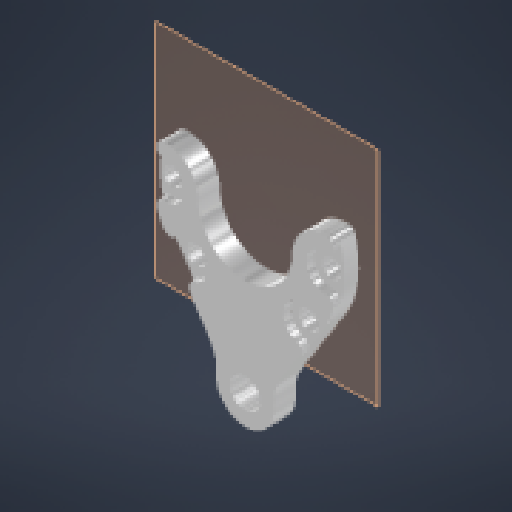
# Autodesk Inventor part: Slider_crank_horn_v2_2025
Saved by Autodesk Inventor 2024.3 (Build 283343000, 343)
## iProperties
Created: 2024-01-23
Part Number: Slider_crank_horn_v2_2025
Material: 알루미늄 6061
Document SubType Name: Modeling
Designer: ASUS
Density: 2.7 g/cm^3
Appearance: 알루미늄 - 평지
Author: ASUS
Autodesk Inventor part; units mm, degrees
(part 1 of 2)
ref_plane "YZ Plane" through (0, 0, 0) normal (1, 0, 0) x (0, 1, 0)
ref_plane "XZ Plane" through (0, 0, 0) normal (0, 1, 0) x (-1, 0, 0)
ref_plane "XY Plane" through (0, 0, 0) normal (0, 0, 1) x (1, 0, 0)
ref_plane "작업 평면1" through (0, 0, 0) normal (0, 0, 1) x (1, 0, 0)
sketch "스케치1" plane through (0, 0, 0) normal (0, 0, 1) x (1, 0, 0)
  circle A0 centre (-11, 0) radius 1.25 projected
  circle A1 centre (11, 0) radius 1.25 projected
  circle A2 centre (7.7782, -7.7782) radius 1.25 projected
  circle A3 centre (-7.7782, 7.7782) radius 1.25 projected
  circle A4 centre (-7.7782, -7.7782) radius 1.25 projected
  circle A5 centre (7.7782, 7.7782) radius 1.25 projected
  circle A6 centre (0, -11) radius 1.25 projected
  circle A7 centre (0, 11) radius 1.25 projected
  circle A8 centre (0, 0) radius 14 projected
  circle A9 centre (0, 0) radius 5 projected
  line L0 (-17, -38.65) -> (-17, -41.35) projected
  line L1 (17, -38.65) -> (17, -41.35) projected
  line L2 (-17, -40) -> (17, -40)
  line L3 (0, -40) -> (0, 0)
  circle A10 centre (0, -20) radius 2.75
  line L4 (-7.7782, -7.7782) -> (0, -20) construction
  line L5 (-11.1527, -9.9258) -> (-3.3746, -22.1476)
  line L6 (3.3746, -17.8524) -> (-4.4036, -5.6305)
  arc A11 (-4.4036, -5.6305) -> (-11.1527, -9.9258) centre (-7.7782, -7.7782) ccw
  arc A12 (-3.3746, -22.1476) -> (3.3746, -17.8524) centre (0, -20) ccw
  line L7 (0, -20) -> (7.7782, -7.7782) construction
  line L8 (-3.3746, -17.8524) -> (4.4036, -5.6305)
  line L9 (11.1527, -9.9258) -> (3.3746, -22.1476)
  arc A13 (-3.3746, -17.8524) -> (3.3746, -22.1476) centre (0, -20) ccw
  arc A14 (11.1527, -9.9258) -> (4.4036, -5.6305) centre (7.7782, -7.7782) ccw
  circle A15 centre (0, 0) radius 7
  circle A16 centre (-7.7782, -7.7782) radius 1.35
  circle A17 centre (0, -11) radius 1.85
  circle A18 centre (7.7782, -7.7782) radius 1.35
  circle A19 centre (0, 0) radius 11
  circle A20 centre (0, 0) radius 9
  circle A21 centre (0, 0) radius 11
  circle A22 centre (0, 0) radius 13
  line L10 (7.7782, -7.7782) -> (0, -20) construction
  line L11 (6.0909, -6.7044) -> (-1.6873, -18.9262)
  line L12 (1.6873, -21.0738) -> (12.1403, -4.6491)
  arc A23 (9.4655, -8.852) -> (6.0909, -6.7044) centre (7.7782, -7.7782) ccw
  arc A24 (-1.6873, -18.9262) -> (1.6873, -21.0738) centre (0, -20) ccw
  line L13 (0, -20) -> (-7.7782, -7.7782) construction
  line L14 (1.6873, -18.9262) -> (-6.0909, -6.7044)
  line L15 (-12.1403, -4.6491) -> (-1.6873, -21.0738)
  arc A25 (-1.6873, -21.0738) -> (1.6873, -18.9262) centre (0, -20) ccw
  arc A26 (-6.0909, -6.7044) -> (-9.4655, -8.852) centre (-7.7782, -7.7782) ccw
  point P0 (-3.8891, -13.8891)
  point P1 (3.8891, -13.8891)
  point P2 (4.9497, -4.9497)
  point P3 (-4.9497, -4.9497)
  point P4 (0.2013, -12.2337)
  point P5 (0, -12.5499)
  point P6 (-0.2013, -12.2337)
  point P7 (3.8891, -13.8891)
  point P8 (-3.8891, -13.8891)
  point P9 (-3.5472, -18.1514)
  point P10 (-3.3746, -22.1476)
  point P11 (3.5472, -18.1514)
  dimension "d0" = 5.5
  dimension "d1" = 8
  dimension "d2" = 2.7
  dimension "d3" = 3.7
  dimension "d4" = 2.7
  dimension "d7" = 2
  dimension "d8" = 2
  dimension "d9" = 2
  dimension "d10" = 4
  dimension "d11" = 4
  constraints: 36 end point, 18 point on circle, 17 tangent, 16 centre point, 8 midpoint, 5 coincident, 4 parallel, 2 collinear, 2 point on line, 1 concentric, 1 vertical, 3 other
  measures "d0" diameter of A10
  measures "d1" diameter of A12
  measures "d2" diameter of A16
  measures "d3" diameter of A17
  measures "d4" diameter of A18
  measures "d8" radial gap between concentric circles of A20 A21
  measures "d9" radial gap between concentric circles of A21 A22
  measures "d10" diameter of A24
  measures "d11" diameter of A26
extrude "돌출1" add sketch "스케치1" along normal blind 5 contours A0 A19 A3 A7 A5 A1 A14 A20 A11 | A0 A19 A11 L15 A22 L12 A14 A1 A5 A7 A3 | A19 A26 L15 A11 | A11 A20 A26 A19 | A26 L14 A19 A16 | A19 A16 L14 A22 L15 A26 | A20 L6 A17 A19 L14 A26 | A14 A19 A23 A20 | A20 L3 A17 L6 | A22 L14 A8 L15 | A20 L8 A17 L3 | A14 L12 A23 A19 | A23 L11 A19 A17 L8 A20 | A23 A19 A18 L11 | A17 L3 A6 L6 | L6 A6 A19 A17 | A19 A17 L8 A22 L14 | A8 L14 L8 A13 L15 | A22 L8 A8 L14 | A17 L8 A6 L3 | A23 L12 A22 L11 A19 A18 | A19 A6 L6 L8 A17 | A8 L8 L14 | L15 A10 L3 A12 A13 | A13 L8 L14 L11 A10 L15 | A22 L3 A8 L8 | L8 A17 L3 A22 | A17 A19 A6 L8 | L11 A22 L6 A17 A19 | L8 L3 A17 | L12 A12 L6 L11 A8 | A8 L11 A22 L12 | A8 L3 L14 L8 | L3 A10 L12 A12 | A22 L6 A8 L3 | L3 A17 L6 A22 | A17 L6 L8 A6 A19 | L11 A8 L6 A22 | A6 L3 L6 | L6 A17 L3 | L3 A6 L8 | L11 L6 A8 | L12 A10 L14 L11 L6 A12 | A8 L6 L11 L3 | L14 A10 L3 | L3 A10 L11
sketch "스케치2" plane through (0, 0, 5) normal (0, 0, 1) x (1, 0, 0)
  circle A0 centre (0, -11) radius 1.25 projected
  circle A1 centre (7.7782, -7.7782) radius 1.35 projected
  circle A2 centre (-11, 0) radius 1.25 projected
  circle A3 centre (-7.7782, -7.7782) radius 1.35 projected
  circle A4 centre (0, -20) radius 2.75 projected
  circle A5 centre (0, 0) radius 9 projected
  circle A6 centre (-7.7782, 7.7782) radius 1.25 projected
  circle A7 centre (0, 11) radius 1.25 projected
  circle A8 centre (7.7782, 7.7782) radius 1.25 projected
  circle A9 centre (11, 0) radius 1.25 projected
  arc A10 (12.1403, -4.6491) -> (-12.1403, -4.6491) centre (0, 0) ccw projected
  line L0 (-12.1403, -4.6491) -> (-3.5472, -18.1514) projected
  arc A11 (-3.5472, -18.1514) -> (3.5472, -18.1514) centre (0, -20) ccw projected
  line L1 (3.5472, -18.1514) -> (12.1403, -4.6491) projected
  circle A12 centre (0, 0) radius 12.7381
  line L2 (3.5472, -18.1514) -> (12.1403, -4.6491) projected
  point P0 (-10.7464, -6.8392)
  point P1 (10.7464, -6.8392)
  constraints: 1 centre point, 1 coincident, 1 tangent
extrude "돌출2" cut sketch "스케치2" against normal through all contours L1 A12 L0 A10
sketch "스케치3" plane through (0, 0, 5) normal (0, 0, 1) x (1, 0, 0)
  circle A0 centre (7.7782, -7.7782) radius 1.35 projected
  circle A1 centre (7.7782, -7.7782) radius 2.5
  circle A2 centre (11, 0) radius 2.5
  circle A3 centre (7.7782, 7.7782) radius 2.5
  circle A4 centre (0, 11) radius 2.5
  circle A5 centre (-7.7782, 7.7782) radius 2.5
  circle A6 centre (-11, 0) radius 2.5
  circle A7 centre (-7.7782, -7.7782) radius 2.5
  circle A8 centre (0, -11) radius 2.5
  point P0 (0, 0)
  dimension "d14" = 5
  dimension "d17" = 360
  constraints: 8 centre point, 1 coincident, 17 other
  measures "d14" diameter of A1
extrude "돌출3" cut sketch "스케치3" against normal blind 2 contours A0 | A1 | A2 | A3 | A4 | A5 | A6 | A7 | A8
fillet "모깎기1" radius 1 30 edges at (5.335, -7.2483, 4) (8.6601, -10.1175, 4) (7.2483, -5.335, 4) (10.2708, -7.5865, 4) (12.5914, -1.9281, 4) (12.5914, 1.9281, 4) (8.8977, 1.3529, 4) (8.8977, -1.3529, 4) (1.3529, -8.8977, 4) (-1.3529, -8.8977, 4) (-5.335, -7.2483, 4) (-7.2483, -5.335, 4) (-8.8977, -1.3529, 4) (-8.6601, -10.1175, 4) (-10.2708, -7.5865, 4) (10.2668, 7.5401, 4) (7.2483, 5.335, 4) (5.335, 7.2483, 4) (7.5401, 10.2668, 4) (1.9281, 12.5914, 4) (-1.3529, 8.8977, 4) (-1.9281, 12.5914, 4) (1.3529, 8.8977, 4) (-5.335, 7.2483, 4) (-7.2483, 5.335, 4) (-7.5401, 10.2668, 4) (-10.2668, 7.5401, 4) (-12.5914, 1.9281, 4) (-8.8977, 1.3529, 4) (-12.5914, -1.9281, 4)
fillet "모깎기2" radius 5 2 edges at (-3.5472, -18.1514, 2.5) (3.5472, -18.1514, 2.5)
sketch "스케치4" plane through (0, 0, 0) normal (0, 0, -1) x (-1, 0, 0)
  arc A0 (10.7464, -6.8392) -> (-10.7464, -6.8392) centre (0, 0) ccw projected
  line L0 (-4.7245, -16.3015) -> (-10.7464, -6.8392) projected
  arc A1 (-3.9745, -19.5493) -> (-4.7245, -16.3015) centre (-8.9427, -18.986) ccw projected
  arc A2 (-3.9745, -19.5493) -> (3.9745, -19.5493) centre (0, -20) ccw projected
  arc A3 (4.7245, -16.3015) -> (3.9745, -19.5493) centre (8.9427, -18.986) ccw projected
  line L1 (10.7464, -6.8392) -> (4.7245, -16.3015) projected
  circle A4 centre (0, -11) radius 1.25 projected
  circle A5 centre (-7.7782, -7.7782) radius 1.35 projected
  circle A6 centre (11, 0) radius 1.25 projected
  circle A7 centre (7.7782, -7.7782) radius 1.35 projected
  circle A8 centre (0, -20) radius 2.75 projected
  circle A9 centre (0, 0) radius 9 projected
  circle A10 centre (7.7782, 7.7782) radius 1.25 projected
  circle A11 centre (0, 11) radius 1.25 projected
  circle A12 centre (-7.7782, 7.7782) radius 1.25 projected
  circle A13 centre (-11, 0) radius 1.25 projected
  circle A14 centre (0, -20) radius 2 projected
  circle A15 centre (0, -20) radius 3 projected
ref_plane "작업 평면2" through (-3.18, -23.18, 4) normal (0, 0, -1) x (-0.0608395, 0.9981476, 0)
extrude "돌출4" add sketch "스케치4" against normal up to surface (4 mm away) contours A8
sketch "스케치5" plane through (0, 0, 0) normal (0, 0, -1) x (-1, 0, 0)
  circle A0 centre (0, -20) radius 2 projected
  arc A1 (10.7464, -6.8392) -> (-10.7464, -6.8392) centre (0, 0) ccw projected
  line L0 (-4.7245, -16.3015) -> (-10.7464, -6.8392) projected
  arc A2 (-3.9745, -19.5493) -> (-4.7245, -16.3015) centre (-8.9427, -18.986) ccw projected
  arc A3 (-3.9745, -19.5493) -> (3.9745, -19.5493) centre (0, -20) ccw projected
  arc A4 (4.7245, -16.3015) -> (3.9745, -19.5493) centre (8.9427, -18.986) ccw projected
  line L1 (10.7464, -6.8392) -> (4.7245, -16.3015) projected
  circle A5 centre (0, -11) radius 1.25 projected
  circle A6 centre (-7.7782, -7.7782) radius 1.35 projected
  circle A7 centre (11, 0) radius 1.25 projected
  circle A8 centre (7.7782, -7.7782) radius 1.35 projected
  circle A9 centre (0, 0) radius 9 projected
  circle A10 centre (7.7782, 7.7782) radius 1.25 projected
  circle A11 centre (0, 11) radius 1.25 projected
  circle A12 centre (-7.7782, 7.7782) radius 1.25 projected
  circle A13 centre (-11, 0) radius 1.25 projected
  circle A14 centre (0, -20) radius 1.75
  dimension "d25" = 3.5
  constraints: 1 centre point, 1 coincident
  measures "d25" diameter of A14
extrude "돌출5" add sketch "스케치5" against normal up to surface (4 mm away) contours A0
sketch "스케치6" plane through (0, 0, 3) normal (0, 0, 1) x (1, 0, 0)
  arc A0 (-4.0295, 8.0475) -> (-8.0475, 4.0295) centre (0, 0) ccw projected
  arc A1 (-5.4204, 8.6093) -> (-4.0295, 8.0475) centre (-4.4772, 8.9417) ccw projected
  arc A2 (-5.4204, 8.6093) -> (-6.1176, 9.647) centre (-7.7782, 7.7782) ccw projected
  arc A3 (-5.9179, 11.28) -> (-6.1176, 9.647) centre (-5.4533, 10.3945) ccw projected
  arc A4 (-5.9179, 11.28) -> (-11.28, 5.9179) centre (0, 0) ccw projected
  arc A5 (-9.647, 6.1176) -> (-11.28, 5.9179) centre (-10.3945, 5.4533) ccw projected
  arc A6 (-9.647, 6.1176) -> (-8.6093, 5.4204) centre (-7.7782, 7.7782) ccw projected
  arc A7 (-8.0475, 4.0295) -> (-8.6093, 5.4204) centre (-8.9417, 4.4772) ccw projected
  circle A8 centre (-7.7782, 7.7782) radius 1.25 projected
  circle A9 centre (0, 11) radius 1.25 projected
  arc A10 (2.8412, 8.5398) -> (-2.8412, 8.5398) centre (0, 0) ccw projected
  arc A11 (2.2549, 9.9205) -> (2.8412, 8.5398) centre (3.1569, 9.4886) ccw projected
  arc A12 (2.2549, 9.9205) -> (2.4957, 11.1472) centre (0, 11) ccw projected
  arc A13 (3.7916, 12.1608) -> (2.4957, 11.1472) centre (3.4939, 11.2061) ccw projected
  arc A14 (3.7916, 12.1608) -> (-3.7916, 12.1608) centre (0, 0) ccw projected
  arc A15 (-2.4957, 11.1472) -> (-3.7916, 12.1608) centre (-3.4939, 11.2061) ccw projected
  arc A16 (-2.4957, 11.1472) -> (-2.2549, 9.9205) centre (0, 11) ccw projected
  arc A17 (-2.8412, 8.5398) -> (-2.2549, 9.9205) centre (-3.1569, 9.4886) ccw projected
  circle A18 centre (7.7782, 7.7782) radius 1.25 projected
  arc A19 (8.0475, 4.0295) -> (4.0295, 8.0475) centre (0, 0) ccw projected
  arc A20 (8.6093, 5.4204) -> (8.0475, 4.0295) centre (8.9417, 4.4772) ccw projected
  arc A21 (8.6093, 5.4204) -> (9.647, 6.1176) centre (7.7782, 7.7782) ccw projected
  arc A22 (11.28, 5.9179) -> (9.647, 6.1176) centre (10.3945, 5.4533) ccw projected
  arc A23 (11.28, 5.9179) -> (5.9179, 11.28) centre (0, 0) ccw projected
  arc A24 (6.1176, 9.647) -> (5.9179, 11.28) centre (5.4533, 10.3945) ccw projected
  arc A25 (6.1176, 9.647) -> (5.4204, 8.6093) centre (7.7782, 7.7782) ccw projected
  arc A26 (4.0295, 8.0475) -> (5.4204, 8.6093) centre (4.4772, 8.9417) ccw projected
  circle A27 centre (11, 0) radius 1.25 projected
  arc A28 (8.5398, -2.8412) -> (8.5398, 2.8412) centre (0, 0) ccw projected
  arc A29 (9.9205, -2.2549) -> (8.5398, -2.8412) centre (9.4886, -3.1569) ccw projected
  arc A30 (9.9205, -2.2549) -> (11.1472, -2.4957) centre (11, 0) ccw projected
  arc A31 (12.1608, -3.7916) -> (11.1472, -2.4957) centre (11.2061, -3.4939) ccw projected
  arc A32 (12.1608, -3.7916) -> (12.1608, 3.7916) centre (0, 0) ccw projected
  arc A33 (11.1472, 2.4957) -> (12.1608, 3.7916) centre (11.2061, 3.4939) ccw projected
  arc A34 (11.1472, 2.4957) -> (9.9205, 2.2549) centre (11, 0) ccw projected
  arc A35 (8.5398, 2.8412) -> (9.9205, 2.2549) centre (9.4886, 3.1569) ccw projected
  arc A36 (4.0295, -8.0475) -> (8.0475, -4.0295) centre (0, 0) ccw projected
  arc A37 (5.4204, -8.6093) -> (4.0295, -8.0475) centre (4.4772, -8.9417) ccw projected
  arc A38 (5.4204, -8.6093) -> (7.0945, -10.1829) centre (7.7782, -7.7782) ccw projected
  arc A39 (7.6646, -11.6816) -> (7.0945, -10.1829) centre (6.821, -11.1447) ccw projected
  line L0 (7.6646, -11.6816) -> (10.7464, -6.8392) projected
  arc A40 (10.7464, -6.8392) -> (11.28, -5.9179) centre (0, 0) ccw projected
  arc A41 (9.647, -6.1176) -> (11.28, -5.9179) centre (10.3945, -5.4533) ccw projected
  arc A42 (9.647, -6.1176) -> (8.6093, -5.4204) centre (7.7782, -7.7782) ccw projected
  arc A43 (8.0475, -4.0295) -> (8.6093, -5.4204) centre (8.9417, -4.4772) ccw projected
  circle A44 centre (7.7782, -7.7782) radius 1.35 projected
  arc A45 (-2.8412, -8.5398) -> (2.8412, -8.5398) centre (0, 0) ccw projected
  arc A46 (-2.2549, -9.9205) -> (-2.8412, -8.5398) centre (-3.1569, -9.4886) ccw projected
  arc A47 (-2.2549, -9.9205) -> (2.2549, -9.9205) centre (0, -11) ccw projected
  arc A48 (2.8412, -8.5398) -> (2.2549, -9.9205) centre (3.1569, -9.4886) ccw projected
  circle A49 centre (0, -11) radius 1.25 projected
  line L1 (-10.7464, -6.8392) -> (-7.6646, -11.6816) projected
  arc A50 (-7.0945, -10.1829) -> (-7.6646, -11.6816) centre (-6.821, -11.1447) ccw projected
  arc A51 (-7.0945, -10.1829) -> (-5.4204, -8.6093) centre (-7.7782, -7.7782) ccw projected
  arc A52 (-4.0295, -8.0475) -> (-5.4204, -8.6093) centre (-4.4772, -8.9417) ccw projected
  arc A53 (-8.0475, -4.0295) -> (-4.0295, -8.0475) centre (0, 0) ccw projected
  arc A54 (-8.6093, -5.4204) -> (-8.0475, -4.0295) centre (-8.9417, -4.4772) ccw projected
  arc A55 (-8.6093, -5.4204) -> (-9.647, -6.1176) centre (-7.7782, -7.7782) ccw projected
  arc A56 (-11.28, -5.9179) -> (-9.647, -6.1176) centre (-10.3945, -5.4533) ccw projected
  arc A57 (-11.28, -5.9179) -> (-10.7464, -6.8392) centre (0, 0) ccw projected
  circle A58 centre (-7.7782, -7.7782) radius 1.35 projected
  arc A59 (-8.5398, 2.8412) -> (-8.5398, -2.8412) centre (0, 0) ccw projected
  arc A60 (-9.9205, 2.2549) -> (-8.5398, 2.8412) centre (-9.4886, 3.1569) ccw projected
  arc A61 (-9.9205, 2.2549) -> (-11.1472, 2.4957) centre (-11, 0) ccw projected
  arc A62 (-12.1608, 3.7916) -> (-11.1472, 2.4957) centre (-11.2061, 3.4939) ccw projected
  arc A63 (-12.1608, 3.7916) -> (-12.1608, -3.7916) centre (0, 0) ccw projected
  arc A64 (-11.1472, -2.4957) -> (-12.1608, -3.7916) centre (-11.2061, -3.4939) ccw projected
  arc A65 (-11.1472, -2.4957) -> (-9.9205, -2.2549) centre (-11, 0) ccw projected
  arc A66 (-8.5398, -2.8412) -> (-9.9205, -2.2549) centre (-9.4886, -3.1569) ccw projected
  circle A67 centre (-11, 0) radius 1.25 projected
extrude "돌출6" cut sketch "스케치6" against normal blind 1 contours A0 A7 A6 A5 A4 A3 A2 A1 | A10 A17 A16 A15 A14 A13 A12 A11 | A19 A26 A25 A24 A23 A22 A21 A20 | A27 | A28 A35 A34 A33 A32 A31 A30 A29 | A36 A43 A42 A41 A40 L0 A39 A38 A37 | A45 A48 A47 A46 | A57 A56 A55 A54 A53 A52 A51 A50 L1 | A59 A66 A65 A64 A63 A62 A61 A60
sketch "스케치7" plane through (0, 0, 5) normal (0, 0, 1) x (1, 0, 0)
  circle A0 centre (0, -20) radius 1.75 projected
  arc A1 (10.7464, -6.8392) -> (-10.7464, -6.8392) centre (0, 0) ccw projected
  line L0 (4.7245, -16.3015) -> (10.7464, -6.8392) projected
  arc A2 (4.7245, -16.3015) -> (3.9745, -19.5493) centre (8.9427, -18.986) ccw projected
  arc A3 (-3.9745, -19.5493) -> (3.9745, -19.5493) centre (0, -20) ccw projected
  arc A4 (-3.9745, -19.5493) -> (-4.7245, -16.3015) centre (-8.9427, -18.986) ccw projected
  line L1 (-10.7464, -6.8392) -> (-4.7245, -16.3015) projected
  circle A5 centre (0, -11) radius 1.25 projected
  circle A6 centre (7.7782, -7.7782) radius 1.35 projected
  circle A7 centre (-11, 0) radius 1.25 projected
  circle A8 centre (-7.7782, -7.7782) radius 1.35 projected
  circle A9 centre (0, 0) radius 9 projected
  circle A10 centre (-7.7782, 7.7782) radius 1.25 projected
  circle A11 centre (0, 11) radius 1.25 projected
  circle A12 centre (7.7782, 7.7782) radius 1.25 projected
  circle A13 centre (11, 0) radius 1.25 projected
  arc A14 (-7.0945, -10.1829) -> (-7.6646, -11.6816) centre (-6.821, -11.1447) ccw projected
  line L2 (-7.6646, -11.6816) -> (-4.7245, -16.3015) projected
  arc A15 (-3.9745, -19.5493) -> (-4.7245, -16.3015) centre (-8.9427, -18.986) ccw projected
  arc A16 (-3.9745, -19.5493) -> (3.9745, -19.5493) centre (0, -20) ccw projected
  arc A17 (4.7245, -16.3015) -> (3.9745, -19.5493) centre (8.9427, -18.986) ccw projected
  line L3 (4.7245, -16.3015) -> (7.6646, -11.6816) projected
  arc A18 (7.6646, -11.6816) -> (7.0945, -10.1829) centre (6.821, -11.1447) ccw projected
  arc A19 (5.4204, -8.6093) -> (7.0945, -10.1829) centre (7.7782, -7.7782) ccw projected
  arc A20 (5.4204, -8.6093) -> (4.0295, -8.0475) centre (4.4772, -8.9417) ccw projected
  arc A21 (2.8412, -8.5398) -> (4.0295, -8.0475) centre (0, 0) ccw projected
  arc A22 (2.8412, -8.5398) -> (2.2549, -9.9205) centre (3.1569, -9.4886) ccw projected
  arc A23 (-2.2549, -9.9205) -> (2.2549, -9.9205) centre (0, -11) ccw projected
  arc A24 (-2.2549, -9.9205) -> (-2.8412, -8.5398) centre (-3.1569, -9.4886) ccw projected
  arc A25 (-4.0295, -8.0475) -> (-2.8412, -8.5398) centre (0, 0) ccw projected
  arc A26 (-4.0295, -8.0475) -> (-5.4204, -8.6093) centre (-4.4772, -8.9417) ccw projected
  arc A27 (-7.0945, -10.1829) -> (-5.4204, -8.6093) centre (-7.7782, -7.7782) ccw projected
  circle A28 centre (0, -20) radius 2.75 projected
  point P0 (-7.6646, -11.6816)
extrude "돌출7" cut sketch "스케치7" against normal up to surface (3 mm away) contours L0 A18 A19 A20 A9 A26 A27 A14 L1 A1
sketch "스케치8" plane through (0, 0, 5) normal (0, 0, 1) x (1, 0, 0)
  circle A0 centre (0, -20) radius 3 projected
  line L0 (-4.4046, -19.0784) -> (-4.3953, -20.9652) projected
  arc A1 (-4.3953, -20.9652) -> (4.4046, -20.9216) centre (0, -20) ccw projected
  line L1 (4.4046, -20.9216) -> (4.3953, -19.0348) projected
  arc A2 (4.3953, -19.0348) -> (-4.4046, -19.0784) centre (0, -20) ccw projected
  arc A3 (-7.0945, -10.1829) -> (-7.6646, -11.6816) centre (-6.821, -11.1447) ccw projected
  line L2 (-7.6646, -11.6816) -> (-4.7245, -16.3015) projected
  arc A4 (-3.9745, -19.5493) -> (-4.7245, -16.3015) centre (-8.9427, -18.986) ccw projected
  arc A5 (-3.9745, -19.5493) -> (3.9745, -19.5493) centre (0, -20) ccw projected
  arc A6 (4.7245, -16.3015) -> (3.9745, -19.5493) centre (8.9427, -18.986) ccw projected
  line L3 (4.7245, -16.3015) -> (7.6646, -11.6816) projected
  arc A7 (7.6646, -11.6816) -> (7.0945, -10.1829) centre (6.821, -11.1447) ccw projected
  arc A8 (5.4204, -8.6093) -> (7.0945, -10.1829) centre (7.7782, -7.7782) ccw projected
  arc A9 (5.4204, -8.6093) -> (4.0295, -8.0475) centre (4.4772, -8.9417) ccw projected
  arc A10 (2.8412, -8.5398) -> (4.0295, -8.0475) centre (0, 0) ccw projected
  arc A11 (2.8412, -8.5398) -> (2.2549, -9.9205) centre (3.1569, -9.4886) ccw projected
  arc A12 (-2.2549, -9.9205) -> (2.2549, -9.9205) centre (0, -11) ccw projected
  arc A13 (-2.2549, -9.9205) -> (-2.8412, -8.5398) centre (-3.1569, -9.4886) ccw projected
  arc A14 (-4.0295, -8.0475) -> (-2.8412, -8.5398) centre (0, 0) ccw projected
  arc A15 (-4.0295, -8.0475) -> (-5.4204, -8.6093) centre (-4.4772, -8.9417) ccw projected
  arc A16 (-7.0945, -10.1829) -> (-5.4204, -8.6093) centre (-7.7782, -7.7782) ccw projected
  circle A17 centre (0, -20) radius 2.75 projected
extrude "돌출8" cut sketch "스케치8" against normal up to surface (1 mm away) contours A0
sketch "스케치9" plane through (0, 0, 2) normal (0, 0, 1) x (1, 0, 0)
  circle A0 centre (11, 0) radius 1.25 projected
  circle A1 centre (-11, 0) radius 1.25 projected
  circle A2 centre (-7.7782, 7.7782) radius 1.25 projected
  circle A3 centre (7.7782, -7.7782) radius 1.25 projected
  circle A4 centre (7.7782, 7.7782) radius 1.25 projected
  circle A5 centre (-7.7782, -7.7782) radius 1.25 projected
  circle A6 centre (0, 11) radius 1.25 projected
  circle A7 centre (0, -11) radius 1.25 projected
  circle A8 centre (0, 0) radius 14 projected
  circle A9 centre (0, 0) radius 5 projected
  circle A10 centre (0, 0) radius 5.5
  circle A11 centre (11, 0) radius 1.25 projected
  circle A12 centre (7.7782, 7.7782) radius 1.25 projected
  circle A13 centre (-7.7782, 7.7782) radius 1.25 projected
  circle A14 centre (0, 11) radius 1.25 projected
  circle A15 centre (-11, 0) radius 1.25 projected
  circle A16 centre (-7.7782, -7.7782) radius 1.35 projected
  arc A17 (7.6646, -11.6816) -> (7.0945, -10.1829) centre (6.821, -11.1447) ccw projected
  line L0 (10.7464, -6.8392) -> (7.6646, -11.6816) projected
  arc A18 (10.7464, -6.8392) -> (-10.7464, -6.8392) centre (0, 0) ccw projected
  line L1 (-7.6646, -11.6816) -> (-10.7464, -6.8392) projected
  arc A19 (-7.0945, -10.1829) -> (-7.6646, -11.6816) centre (-6.821, -11.1447) ccw projected
  arc A20 (-7.0945, -10.1829) -> (-5.4204, -8.6093) centre (-7.7782, -7.7782) ccw projected
  arc A21 (-4.0295, -8.0475) -> (-5.4204, -8.6093) centre (-4.4772, -8.9417) ccw projected
  arc A22 (4.0295, -8.0475) -> (-4.0295, -8.0475) centre (0, 0) ccw projected
  arc A23 (5.4204, -8.6093) -> (4.0295, -8.0475) centre (4.4772, -8.9417) ccw projected
  arc A24 (5.4204, -8.6093) -> (7.0945, -10.1829) centre (7.7782, -7.7782) ccw projected
  circle A25 centre (7.7782, -7.7782) radius 1.35 projected
  circle A26 centre (0, -20) radius 1.75 projected
  arc A27 (10.7464, -6.8392) -> (-10.7464, -6.8392) centre (0, 0) ccw projected
  line L2 (4.7245, -16.3015) -> (10.7464, -6.8392) projected
  arc A28 (4.7245, -16.3015) -> (3.9745, -19.5493) centre (8.9427, -18.986) ccw projected
  arc A29 (-3.9745, -19.5493) -> (3.9745, -19.5493) centre (0, -20) ccw projected
  arc A30 (-3.9745, -19.5493) -> (-4.7245, -16.3015) centre (-8.9427, -18.986) ccw projected
  line L3 (-10.7464, -6.8392) -> (-4.7245, -16.3015) projected
  circle A31 centre (0, -11) radius 1.25 projected
  circle A32 centre (7.7782, -7.7782) radius 1.35 projected
  circle A33 centre (-11, 0) radius 1.25 projected
  circle A34 centre (-7.7782, -7.7782) radius 1.35 projected
  circle A35 centre (0, 0) radius 9 projected
  circle A36 centre (-7.7782, 7.7782) radius 1.25 projected
  circle A37 centre (0, 11) radius 1.25 projected
  circle A38 centre (7.7782, 7.7782) radius 1.25 projected
  circle A39 centre (11, 0) radius 1.25 projected
  point P0 (-4.0295, -8.0475)
  dimension "d34" = 0.5
  constraints: 1 centre point
  measures "d34" radial gap between concentric circles of A9 A10
extrude "돌출9" add sketch "스케치9" against normal up to surface (2 mm away) contours A22 A35
sketch "스케치10" plane through (0, -20, 4) normal (0, 0, 1) x (1, 0, 0)
  circle A0 centre (0, 0) radius 3 projected
  circle A1 centre (0, 0) radius 1.75 projected
  circle A2 centre (0, 0) radius 2.03
  point P0 (0, 20)
  dimension "d37" = 4.06
  constraints: 1 centre point, 1 coincident
  measures "d37" diameter of A2
extrude "돌출10" cut sketch "스케치10" against normal through all contours A1 | A2
sketch "스케치11" plane through (0, 0, 5) normal (0, 0, 1) x (1, 0, 0)
  circle A0 centre (0, -20) radius 2.03 projected
  circle A1 centre (0, -20) radius 3 projected
  point P0 (0, 0)
extrude "돌출11" add sketch "스케치11" against normal up to surface (1 mm away)
sketch "스케치12" plane through (0, 0, 0) normal (0, 0, -1) x (-1, 0, 0)
  line L0 (10.9195, -14.3086) -> (12.3787, -15.1511)
  arc A0 (13.3991, -16.9184) -> (12.3787, -15.1511) centre (12.5331, -16.2402) ccw
  line L1 (13.3991, -16.9184) -> (13.3991, -18.6034)
  arc A1 (12.3787, -20.3708) -> (13.3991, -18.6034) centre (12.5331, -19.2816) ccw
  line L2 (12.3787, -20.3708) -> (10.9195, -21.2133)
  arc A2 (8.8787, -21.2133) -> (10.9195, -21.2133) centre (9.8991, -20.8024) ccw
  line L3 (8.8787, -21.2133) -> (7.4195, -20.3708)
  arc A3 (6.3991, -18.6034) -> (7.4195, -20.3708) centre (7.2651, -19.2816) ccw
  line L4 (6.3991, -18.6034) -> (6.3991, -16.9184)
  arc A4 (7.4195, -15.1511) -> (6.3991, -16.9184) centre (7.2651, -16.2402) ccw
  line L5 (7.4195, -15.1511) -> (8.8787, -14.3086)
  arc A5 (10.9195, -14.3086) -> (8.8787, -14.3086) centre (9.8991, -14.7195) ccw
  arc A6 (14.5658, -19.556) -> (13.8991, -23.1461) centre (23.8991, -23.1461) ccw
  arc A7 (14.5658, -19.556) -> (5.2324, -19.556) centre (9.8991, -17.7609) ccw
  arc A8 (5.8991, -23.1461) -> (5.2324, -19.556) centre (-4.1009, -23.1461) ccw
  circle A9 centre (0, -20) radius 2.03 projected
  circle A10 centre (0, 0) radius 5.5 projected
  arc A11 (10.7464, -6.8392) -> (-10.7464, -6.8392) centre (0, 0) ccw projected
  line L6 (-4.7245, -16.3015) -> (-10.7464, -6.8392) projected
  arc A12 (-3.9745, -19.5493) -> (-4.7245, -16.3015) centre (-8.9427, -18.986) ccw projected
  arc A13 (-3.9745, -19.5493) -> (3.9745, -19.5493) centre (0, -20) ccw projected
  arc A14 (4.7245, -16.3015) -> (3.9745, -19.5493) centre (8.9427, -18.986) ccw projected
  line L7 (10.7464, -6.8392) -> (4.7245, -16.3015) projected
  circle A15 centre (0, -11) radius 1.25 projected
  circle A16 centre (-7.7782, -7.7782) radius 1.35 projected
  circle A17 centre (11, 0) radius 1.25 projected
  circle A18 centre (7.7782, -7.7782) radius 1.35 projected
  circle A19 centre (7.7782, 7.7782) radius 1.25 projected
  circle A20 centre (0, 11) radius 1.25 projected
  circle A21 centre (-7.7782, 7.7782) radius 1.25 projected
  circle A22 centre (-11, 0) radius 1.25 projected
  arc A23 (3.5, -19.1575) -> (2.4796, -17.3902) centre (2.634, -18.4793) ccw
  arc A24 (1.0204, -16.5477) -> (-1.0204, -16.5477) centre (0, -16.9585) ccw
  line L8 (3.5, -19.1575) -> (3.5, -20.8425)
  line L9 (-2.4796, -17.3902) -> (-1.0204, -16.5477)
  arc A25 (2.4796, -22.6098) -> (3.5, -20.8425) centre (2.634, -21.5207) ccw
  line L10 (2.4796, -22.6098) -> (1.0204, -23.4523)
  arc A26 (4.6667, -21.7951) -> (-4.6667, -21.7951) centre (0, -20) ccw
  arc A27 (-1.0204, -23.4523) -> (1.0204, -23.4523) centre (0, -23.0415) ccw
  line L11 (-3.5, -20.8425) -> (-3.5, -19.1575)
  line L12 (-1.0204, -23.4523) -> (-2.4796, -22.6098)
  arc A28 (-3.5, -20.8425) -> (-2.4796, -22.6098) centre (-2.634, -21.5207) ccw
  arc A29 (-4, -25.3852) -> (-4.6667, -21.7951) centre (-14, -25.3852) ccw
  arc A30 (-2.4796, -17.3902) -> (-3.5, -19.1575) centre (-2.634, -18.4793) ccw
  line L13 (1.0204, -16.5477) -> (2.4796, -17.3902)
  arc A31 (4.6667, -21.7951) -> (4, -25.3852) centre (14, -25.3852) ccw
  constraints: 36 point on circle, 24 end point, 18 centre point
ref_plane "작업 평면3" through (-3.5, -24.0415, 3) normal (0, 0, 1) x (1, 0, 0)
extrude "돌출12" cut sketch "스케치12" against normal up to surface (3 mm away) contours A9 | A25 A13 | A13 A25 L10 A27 L12 A28 L11 A30 L9 A24 L13 A23 L8 | A13 A28 | A27 A13
sketch "스케치13" plane through (0, 0, 2) normal (0, 0, 1) x (1, 0, 0)
  circle A0 centre (0, -20) radius 2.03 projected
  arc A1 (-7.0945, -10.1829) -> (-7.6646, -11.6816) centre (-6.821, -11.1447) ccw projected
  line L0 (-7.6646, -11.6816) -> (-4.7245, -16.3015) projected
  arc A2 (-3.9745, -19.5493) -> (-4.7245, -16.3015) centre (-8.9427, -18.986) ccw projected
  arc A3 (-3.9745, -19.5493) -> (3.9745, -19.5493) centre (0, -20) ccw projected
  arc A4 (4.7245, -16.3015) -> (3.9745, -19.5493) centre (8.9427, -18.986) ccw projected
  line L1 (4.7245, -16.3015) -> (7.6646, -11.6816) projected
  arc A5 (7.6646, -11.6816) -> (7.0945, -10.1829) centre (6.821, -11.1447) ccw projected
  arc A6 (5.4204, -8.6093) -> (7.0945, -10.1829) centre (7.7782, -7.7782) ccw projected
  arc A7 (5.4204, -8.6093) -> (4.0295, -8.0475) centre (4.4772, -8.9417) ccw projected
  arc A8 (2.8412, -8.5398) -> (4.0295, -8.0475) centre (0, 0) ccw projected
  arc A9 (2.8412, -8.5398) -> (2.2549, -9.9205) centre (3.1569, -9.4886) ccw projected
  arc A10 (-2.2549, -9.9205) -> (2.2549, -9.9205) centre (0, -11) ccw projected
  arc A11 (-2.2549, -9.9205) -> (-2.8412, -8.5398) centre (-3.1569, -9.4886) ccw projected
  arc A12 (-4.0295, -8.0475) -> (-2.8412, -8.5398) centre (0, 0) ccw projected
  arc A13 (-4.0295, -8.0475) -> (-5.4204, -8.6093) centre (-4.4772, -8.9417) ccw projected
  arc A14 (-7.0945, -10.1829) -> (-5.4204, -8.6093) centre (-7.7782, -7.7782) ccw projected
  circle A15 centre (7.7782, -7.7782) radius 1.35 projected
  circle A16 centre (-7.7782, -7.7782) radius 1.35 projected
  circle A17 centre (-11, 0) radius 1.25 projected
  circle A18 centre (0, 11) radius 1.25 projected
  circle A19 centre (-7.7782, 7.7782) radius 1.25 projected
  circle A20 centre (7.7782, 7.7782) radius 1.25 projected
  circle A21 centre (11, 0) radius 1.25 projected
  circle A22 centre (0, 0) radius 5.5 projected
  arc A23 (2.8412, -8.5398) -> (2.2549, -9.9205) centre (3.1569, -9.4886) ccw projected
  arc A24 (2.8412, -8.5398) -> (4.0295, -8.0475) centre (0, 0) ccw projected
  arc A25 (5.4204, -8.6093) -> (4.0295, -8.0475) centre (4.4772, -8.9417) ccw projected
  arc A26 (5.4204, -8.6093) -> (7.0945, -10.1829) centre (7.7782, -7.7782) ccw projected
  arc A27 (7.6646, -11.6816) -> (7.0945, -10.1829) centre (6.821, -11.1447) ccw projected
  line L2 (10.7464, -6.8392) -> (7.6646, -11.6816) projected
  arc A28 (10.7464, -6.8392) -> (-10.7464, -6.8392) centre (0, 0) ccw projected
  line L3 (-7.6646, -11.6816) -> (-10.7464, -6.8392) projected
  arc A29 (-7.0945, -10.1829) -> (-7.6646, -11.6816) centre (-6.821, -11.1447) ccw projected
  arc A30 (-7.0945, -10.1829) -> (-5.4204, -8.6093) centre (-7.7782, -7.7782) ccw projected
  arc A31 (-4.0295, -8.0475) -> (-5.4204, -8.6093) centre (-4.4772, -8.9417) ccw projected
  arc A32 (-4.0295, -8.0475) -> (-2.8412, -8.5398) centre (0, 0) ccw projected
  arc A33 (-2.2549, -9.9205) -> (-2.8412, -8.5398) centre (-3.1569, -9.4886) ccw projected
  arc A34 (-2.2549, -9.9205) -> (2.2549, -9.9205) centre (0, -11) ccw projected
  circle A35 centre (0, -11) radius 1.25 projected
  point P0 (-7.6646, -11.6816)
extrude "돌출13" add sketch "스케치13" along normal up to surface (3 mm away) contours A1 L3 A28 L2 A5 A6 A7 A8 A9 A10 A11 A12 A13 A14
sketch "스케치14" plane through (0, 0, 5) normal (0, 0, 1) x (1, 0, 0)
  circle A0 centre (0, -11) radius 1.25 projected
  circle A1 centre (0, 0) radius 5.5 projected
  circle A2 centre (11, 0) radius 1.25 projected
  circle A3 centre (7.7782, 7.7782) radius 1.25 projected
  circle A4 centre (-7.7782, 7.7782) radius 1.25 projected
  circle A5 centre (0, 11) radius 1.25 projected
  circle A6 centre (-11, 0) radius 1.25 projected
  circle A7 centre (-7.7782, -7.7782) radius 1.35 projected
  circle A8 centre (7.7782, -7.7782) radius 1.35 projected
  circle A9 centre (0, -20) radius 2.03 projected
  line L0 (4.7245, -16.3015) -> (10.7464, -6.8392) projected
  arc A10 (10.7464, -6.8392) -> (-10.7464, -6.8392) centre (0, 0) ccw projected
  line L1 (-10.7464, -6.8392) -> (-4.7245, -16.3015) projected
  arc A11 (-3.9745, -19.5493) -> (-4.7245, -16.3015) centre (-8.9427, -18.986) ccw projected
  arc A12 (-3.9745, -19.5493) -> (3.9745, -19.5493) centre (0, -20) ccw projected
  arc A13 (4.7245, -16.3015) -> (3.9745, -19.5493) centre (8.9427, -18.986) ccw projected
  circle A14 centre (-11, 0) radius 2.5
  circle A15 centre (-7.7782, 7.7782) radius 2.5
  circle A16 centre (0, 11) radius 2.5
  circle A17 centre (7.7782, 7.7782) radius 2.5
  circle A18 centre (11, 0) radius 2.5
  circle A19 centre (-7.7782, -7.7782) radius 2.5
  circle A20 centre (0, -11) radius 2.5
  circle A21 centre (7.7782, -7.7782) radius 2.5
  dimension "d46" = 5
  dimension "d47" = 5
  dimension "d48" = 5
  dimension "d49" = 5
  dimension "d50" = 5
  dimension "d51" = 5
  dimension "d52" = 5
  dimension "d53" = 5
  constraints: 8 centre point, 8 coincident
  measures "d46" diameter of A14
  measures "d47" diameter of A15
  measures "d48" diameter of A16
  measures "d49" diameter of A17
  measures "d50" diameter of A18
  measures "d51" diameter of A19
  measures "d52" diameter of A20
  measures "d53" diameter of A21
extrude "돌출14" cut sketch "스케치14" against normal blind 3 contours A2 | A3 | A4 | A5 | A6 | A7 | A8 | A21 L0 | L0 A21 | A18 A10 | A10 A18 | A19 L1 | L1 A19 | A17 A10 | A10 A17 | A14 A10 | A10 A14 | A16 A10 | A10 A16 | A15 A10 | A10 A15 | A20
sketch "스케치15" plane through (0, 0, 5) normal (0, 0, 1) x (1, 0, 0)
  circle A0 centre (0, -20) radius 2.03 projected
  circle A1 centre (0, 0) radius 5.5 projected
  circle A2 centre (0, -11) radius 2.5 projected
  arc A3 (-1.9281, 12.5914) -> (1.9281, 12.5914) centre (0, 11) ccw projected
  arc A4 (-1.9281, 12.5914) -> (-7.5401, 10.2668) centre (0, 0) ccw projected
  arc A5 (-10.2668, 7.5401) -> (-7.5401, 10.2668) centre (-7.7782, 7.7782) ccw projected
  arc A6 (-10.2668, 7.5401) -> (-12.5914, 1.9281) centre (0, 0) ccw projected
  arc A7 (-12.5914, -1.9281) -> (-12.5914, 1.9281) centre (-11, 0) ccw projected
  arc A8 (-12.5914, -1.9281) -> (-10.7464, -6.8392) centre (0, 0) ccw projected
  line L0 (-10.7464, -6.8392) -> (-10.2708, -7.5865) projected
  arc A9 (-8.6601, -10.1175) -> (-10.2708, -7.5865) centre (-7.7782, -7.7782) ccw projected
  line L1 (-8.6601, -10.1175) -> (-4.7245, -16.3015) projected
  arc A10 (-3.9745, -19.5493) -> (-4.7245, -16.3015) centre (-8.9427, -18.986) ccw projected
  arc A11 (-3.9745, -19.5493) -> (3.9745, -19.5493) centre (0, -20) ccw projected
  arc A12 (4.7245, -16.3015) -> (3.9745, -19.5493) centre (8.9427, -18.986) ccw projected
  line L2 (4.7245, -16.3015) -> (8.6601, -10.1175) projected
  arc A13 (10.2708, -7.5865) -> (8.6601, -10.1175) centre (7.7782, -7.7782) ccw projected
  line L3 (10.2708, -7.5865) -> (10.7464, -6.8392) projected
  arc A14 (10.7464, -6.8392) -> (12.5914, -1.9281) centre (0, 0) ccw projected
  arc A15 (12.5914, 1.9281) -> (12.5914, -1.9281) centre (11, 0) ccw projected
  arc A16 (12.5914, 1.9281) -> (10.2668, 7.5401) centre (0, 0) ccw projected
  arc A17 (7.5401, 10.2668) -> (10.2668, 7.5401) centre (7.7782, 7.7782) ccw projected
  arc A18 (7.5401, 10.2668) -> (1.9281, 12.5914) centre (0, 0) ccw projected
  circle A19 centre (-11, 0) radius 1.25 projected
  circle A20 centre (-11, 0) radius 4
  circle A21 centre (11, 0) radius 4
  circle A22 centre (0, 0) radius 7
  arc A23 (-7.5401, 10.2668) -> (-10.2668, 7.5401) centre (0, 0) ccw projected
  arc A24 (-10.2668, 7.5401) -> (-7.5401, 10.2668) centre (-7.7782, 7.7782) ccw projected
  circle A25 centre (-7.7782, 7.7782) radius 1.25 projected
  arc A26 (1.9281, 12.5914) -> (-1.9281, 12.5914) centre (0, 0) ccw projected
  arc A27 (-1.9281, 12.5914) -> (1.9281, 12.5914) centre (0, 11) ccw projected
  circle A28 centre (0, 11) radius 1.25 projected
  arc A29 (10.2668, 7.5401) -> (7.5401, 10.2668) centre (0, 0) ccw projected
  arc A30 (7.5401, 10.2668) -> (10.2668, 7.5401) centre (7.7782, 7.7782) ccw projected
  circle A31 centre (7.7782, 7.7782) radius 1.25 projected
  point P0 (-12.1482, 3.8317)
  point P1 (-7, 0)
  point P2 (7, 0)
  point P3 (12.1482, 3.8317)
  point P4 (10.2668, 7.5401)
  point P5 (7.5401, 10.2668)
  point P6 (1.9281, 12.5914)
  point P7 (-1.9281, 12.5914)
  point P8 (-7.5401, 10.2668)
  dimension "d56" = 8
  dimension "d57" = 8
  constraints: 3 centre point, 3 coincident, 1 tangent
  measures "d56" diameter of A20
  measures "d57" diameter of A21
extrude "돌출15" cut sketch "스케치15" along normal blind 5 and the other way blind 5 contours A26 A3 | A3 A18 A17 A16 A21 A22 A20 A6 A5 A4 | A5 A23 | A29 A17
sketch "스케치16" plane through (0, 0, 5) normal (0, 0, 1) x (1, 0, 0)
  arc A0 (-7, 0) -> (-12.1482, 3.8317) centre (-11, 0) ccw projected
  arc A1 (-12.1482, 3.8317) -> (-12.5914, 1.9281) centre (0, 0) ccw projected
  arc A2 (-12.5914, -1.9281) -> (-12.5914, 1.9281) centre (-11, 0) ccw projected
  arc A3 (-12.5914, -1.9281) -> (-10.7464, -6.8392) centre (0, 0) ccw projected
  line L0 (-10.7464, -6.8392) -> (-10.2708, -7.5865) projected
  arc A4 (-8.6601, -10.1175) -> (-10.2708, -7.5865) centre (-7.7782, -7.7782) ccw projected
  line L1 (-8.6601, -10.1175) -> (-4.7245, -16.3015) projected
  arc A5 (-3.9745, -19.5493) -> (-4.7245, -16.3015) centre (-8.9427, -18.986) ccw projected
  arc A6 (-3.9745, -19.5493) -> (3.9745, -19.5493) centre (0, -20) ccw projected
  arc A7 (4.7245, -16.3015) -> (3.9745, -19.5493) centre (8.9427, -18.986) ccw projected
  line L2 (4.7245, -16.3015) -> (8.6601, -10.1175) projected
  arc A8 (10.2708, -7.5865) -> (8.6601, -10.1175) centre (7.7782, -7.7782) ccw projected
  line L3 (10.2708, -7.5865) -> (10.7464, -6.8392) projected
  arc A9 (10.7464, -6.8392) -> (12.5914, -1.9281) centre (0, 0) ccw projected
  arc A10 (12.5914, 1.9281) -> (12.5914, -1.9281) centre (11, 0) ccw projected
  arc A11 (12.5914, 1.9281) -> (12.1482, 3.8317) centre (0, 0) ccw projected
  arc A12 (12.1482, 3.8317) -> (7, 0) centre (11, 0) ccw projected
  arc A13 (7, 0) -> (-7, 0) centre (0, 0) ccw projected
  circle A14 centre (0, -20) radius 2.03 projected
  circle A15 centre (0, 0) radius 5.5 projected
  circle A16 centre (0, -11) radius 2.5 projected
  circle A17 centre (0, 0) radius 7
  constraints: 1 centre point, 1 coincident
extrude "돌출16" cut sketch "스케치16" against normal through all contours A13 A17
sketch "스케치17" plane through (0, 0, 5) normal (0, 0, 1) x (1, 0, 0)
  circle A0 centre (0, -11) radius 2.5 projected
  circle A1 centre (0, -20) radius 2.03 projected
  arc A2 (-7, 0) -> (7, 0) centre (0, 0) ccw projected
  arc A3 (-7, 0) -> (-12.1482, 3.8317) centre (-11, 0) ccw projected
  arc A4 (-12.1482, 3.8317) -> (-12.5914, 1.9281) centre (0, 0) ccw projected
  arc A5 (-12.5914, -1.9281) -> (-12.5914, 1.9281) centre (-11, 0) ccw projected
  arc A6 (-12.5914, -1.9281) -> (-10.7464, -6.8392) centre (0, 0) ccw projected
  line L0 (-10.7464, -6.8392) -> (-10.2708, -7.5865) projected
  arc A7 (-8.6601, -10.1175) -> (-10.2708, -7.5865) centre (-7.7782, -7.7782) ccw projected
  line L1 (-8.6601, -10.1175) -> (-4.7245, -16.3015) projected
  arc A8 (-3.9745, -19.5493) -> (-4.7245, -16.3015) centre (-8.9427, -18.986) ccw projected
  arc A9 (-3.9745, -19.5493) -> (3.9745, -19.5493) centre (0, -20) ccw projected
  arc A10 (4.7245, -16.3015) -> (3.9745, -19.5493) centre (8.9427, -18.986) ccw projected
  line L2 (4.7245, -16.3015) -> (8.6601, -10.1175) projected
  arc A11 (10.2708, -7.5865) -> (8.6601, -10.1175) centre (7.7782, -7.7782) ccw projected
  line L3 (10.2708, -7.5865) -> (10.7464, -6.8392) projected
  arc A12 (10.7464, -6.8392) -> (12.5914, -1.9281) centre (0, 0) ccw projected
  arc A13 (12.5914, 1.9281) -> (12.5914, -1.9281) centre (11, 0) ccw projected
  arc A14 (12.5914, 1.9281) -> (12.1482, 3.8317) centre (0, 0) ccw projected
  arc A15 (12.1482, 3.8317) -> (7, 0) centre (11, 0) ccw projected
extrude "돌출17" cut sketch "스케치17" against normal through all contours A0
sketch "스케치18" plane through (0, -16.9585, 3) normal (0, 0, -1) x (-1, 0, 0)
  circle A0 centre (0, -3.0415) radius 2.03 projected
  arc A1 (3.1142, -5.5518) -> (3.7311, -4.4832) centre (0, -3.0415) ccw projected
  arc A2 (3.7311, -4.4832) -> (3.5, -3.8839) centre (2.634, -4.5622) ccw projected
  line L0 (3.5, -3.8839) -> (3.5, -2.199) projected
  arc A3 (3.5, -2.199) -> (2.4796, -0.4316) centre (2.634, -1.5207) ccw projected
  line L1 (2.4796, -0.4316) -> (1.0204, 0.4109) projected
  arc A4 (1.0204, 0.4109) -> (-1.0204, 0.4109) centre (0, 0) ccw projected
  line L2 (-1.0204, 0.4109) -> (-2.4796, -0.4316) projected
  arc A5 (-2.4796, -0.4316) -> (-3.5, -2.199) centre (-2.634, -1.5207) ccw projected
  line L3 (-3.5, -2.199) -> (-3.5, -3.8839) projected
  arc A6 (-3.5, -3.8839) -> (-3.7311, -4.4832) centre (-2.634, -4.5622) ccw projected
  arc A7 (-3.7311, -4.4832) -> (-3.1142, -5.5518) centre (0, -3.0415) ccw projected
  arc A8 (-3.1142, -5.5518) -> (-2.4796, -5.6513) centre (-2.634, -4.5622) ccw projected
  line L4 (-2.4796, -5.6513) -> (-1.0204, -6.4938) projected
  arc A9 (-1.0204, -6.4938) -> (-0.617, -6.9936) centre (0, -6.0829) ccw projected
  arc A10 (-0.617, -6.9936) -> (0.617, -6.9936) centre (0, -3.0415) ccw projected
  arc A11 (0.617, -6.9936) -> (1.0204, -6.4938) centre (0, -6.0829) ccw projected
  line L5 (1.0204, -6.4938) -> (2.4796, -5.6513) projected
  arc A12 (2.4796, -5.6513) -> (3.1142, -5.5518) centre (2.634, -4.5622) ccw projected
  point P0 (0, 16.9585)
extrude "돌출18" add sketch "스케치18" along normal up to surface (3 mm away)
sketch "스케치19" plane through (0, 0, 0) normal (0, 0, -1) x (-1, 0, 0)
  circle A0 centre (0, -20) radius 2.03 projected
  circle A1 centre (0, -20) radius 2.05
  point P0 (0, 0)
  dimension "d68" = 4.1
  constraints: 1 centre point, 1 coincident
  measures "d68" diameter of A1
extrude "돌출19" cut sketch "스케치19" against normal through all contours A0 | A1
sketch "스케치20" plane through (0, 0, 5) normal (0, 0, 1) x (1, 0, 0)
  circle A0 centre (0, -20) radius 2.05 projected
  circle A1 centre (0, -11) radius 2.5 projected
  arc A2 (-7, 0) -> (7, 0) centre (0, 0) ccw projected
  arc A3 (-7, 0) -> (-12.1482, 3.8317) centre (-11, 0) ccw projected
  arc A4 (-12.1482, 3.8317) -> (-12.5914, 1.9281) centre (0, 0) ccw projected
  arc A5 (-12.5914, -1.9281) -> (-12.5914, 1.9281) centre (-11, 0) ccw projected
  arc A6 (-12.5914, -1.9281) -> (-10.7464, -6.8392) centre (0, 0) ccw projected
  line L0 (-10.7464, -6.8392) -> (-10.2708, -7.5865) projected
  arc A7 (-8.6601, -10.1175) -> (-10.2708, -7.5865) centre (-7.7782, -7.7782) ccw projected
  line L1 (-8.6601, -10.1175) -> (-4.7245, -16.3015) projected
  arc A8 (-3.9745, -19.5493) -> (-4.7245, -16.3015) centre (-8.9427, -18.986) ccw projected
  arc A9 (-3.9745, -19.5493) -> (3.9745, -19.5493) centre (0, -20) ccw projected
  arc A10 (4.7245, -16.3015) -> (3.9745, -19.5493) centre (8.9427, -18.986) ccw projected
  line L2 (4.7245, -16.3015) -> (8.6601, -10.1175) projected
  arc A11 (10.2708, -7.5865) -> (8.6601, -10.1175) centre (7.7782, -7.7782) ccw projected
  line L3 (10.2708, -7.5865) -> (10.7464, -6.8392) projected
  arc A12 (10.7464, -6.8392) -> (12.5914, -1.9281) centre (0, 0) ccw projected
  arc A13 (12.5914, 1.9281) -> (12.5914, -1.9281) centre (11, 0) ccw projected
  arc A14 (12.5914, 1.9281) -> (12.1482, 3.8317) centre (0, 0) ccw projected
  arc A15 (12.1482, 3.8317) -> (7, 0) centre (11, 0) ccw projected
  circle A16 centre (0, -20) radius 4
  circle A17 centre (0, -11) radius 2.5 projected
  line L4 (-2.4969, -11.125) -> (-2.0474, -20.1025)
  line L5 (2.045, -20.1514) -> (2.4969, -11.125)
  circle A18 centre (0, -20) radius 2.05 projected
  circle A19 centre (0, -20) radius 3.5
  point P0 (2.4969, -11.125)
  point P1 (-2.1893, -17.2692)
  point P2 (2.1893, -17.2692)
  dimension "d71" = 7
  constraints: 4 end point, 4 tangent, 2 centre point, 2 coincident, 2 point on circle, 3 other
  measures "d71" diameter of A19
extrude "돌출20" cut sketch "스케치20" against normal through all contours L4 A16 L5 A19 | L4 A1 L5 A16
fillet "모깎기3" radius 1 2 edges at (-2.1893, -17.2692, 2.5) (2.1893, -17.2692, 2.5)
fillet "모깎기4" radius 1 12 edges at (-12.1482, 3.8317, 1) (-12.1482, 3.8317, 3.5) (12.1482, 3.8317, 1) (12.1482, 3.8317, 3.5) (12.5914, 1.9281, 3.5) (12.5914, -1.9281, 3.5) (10.2708, -7.5865, 3.5) (8.6601, -10.1175, 3.5) (-8.6601, -10.1175, 3.5) (-10.2708, -7.5865, 3.5) (-12.5914, -1.9281, 3.5) (-12.5914, 1.9281, 3.5)
sketch "스케치22" plane through (0, 0, 5) normal (0, 0, 1) x (1, 0, 0)
  arc A0 (-12.3211, 3.2329) -> (-11.2519, 2.4873) centre (-11.3527, 3.4822) ccw projected
  circle A1 centre (-11.3527, 3.4822) radius 1
  arc A2 (11.2519, 2.4873) -> (12.3211, 3.2329) centre (11.3527, 3.4822) ccw projected
  circle A3 centre (11.3527, 3.4822) radius 1
  arc A4 (-12.3211, 3.2329) -> (-11.2519, 2.4873) centre (-11.3527, 3.4822) ccw projected
  arc A5 (-11.1472, -2.4957) -> (-11.2519, 2.4873) centre (-11, 0) ccw projected
  arc A6 (-11.1472, -2.4957) -> (-12.1608, -3.7916) centre (-11.2061, -3.4939) ccw projected
  arc A7 (-12.1608, -3.7916) -> (-11.28, -5.9179) centre (0, 0) ccw projected
  arc A8 (-11.28, -5.9179) -> (-9.647, -6.1176) centre (-10.3945, -5.4533) ccw projected
  arc A9 (-7.0945, -10.1829) -> (-9.647, -6.1176) centre (-7.7782, -7.7782) ccw projected
  arc A10 (-7.0945, -10.1829) -> (-7.6646, -11.6816) centre (-6.821, -11.1447) ccw projected
  line L0 (-7.6646, -11.6816) -> (-4.7245, -16.3015) projected
  arc A11 (-3.9745, -19.5493) -> (-4.7245, -16.3015) centre (-8.9427, -18.986) ccw projected
  arc A12 (-3.9745, -19.5493) -> (3.9745, -19.5493) centre (0, -20) ccw projected
  arc A13 (4.7245, -16.3015) -> (3.9745, -19.5493) centre (8.9427, -18.986) ccw projected
  line L1 (4.7245, -16.3015) -> (7.6646, -11.6816) projected
  arc A14 (7.6646, -11.6816) -> (7.0945, -10.1829) centre (6.821, -11.1447) ccw projected
  arc A15 (9.647, -6.1176) -> (7.0945, -10.1829) centre (7.7782, -7.7782) ccw projected
  arc A16 (9.647, -6.1176) -> (11.28, -5.9179) centre (10.3945, -5.4533) ccw projected
  arc A17 (11.28, -5.9179) -> (12.1608, -3.7916) centre (0, 0) ccw projected
  arc A18 (12.1608, -3.7916) -> (11.1472, -2.4957) centre (11.2061, -3.4939) ccw projected
  arc A19 (11.2519, 2.4873) -> (11.1472, -2.4957) centre (11, 0) ccw projected
  arc A20 (11.2519, 2.4873) -> (12.3211, 3.2329) centre (11.3527, 3.4822) ccw projected
  arc A21 (12.3211, 3.2329) -> (11.4718, 3.9721) centre (11.3538, 2.9791) ccw projected
  arc A22 (11.4718, 3.9721) -> (7, 0) centre (11, 0) ccw projected
  arc A23 (-7, 0) -> (7, 0) centre (0, 0) ccw projected
  arc A24 (-7, 0) -> (-11.4718, 3.9721) centre (-11, 0) ccw projected
  arc A25 (-11.4718, 3.9721) -> (-12.3211, 3.2329) centre (-11.3538, 2.9791) ccw projected
  circle A26 centre (0, -20) radius 2.05 projected
  line L2 (2.4969, -11.125) -> (2.2662, -15.7322) projected
  arc A27 (0.9858, -16.6417) -> (2.2662, -15.7322) centre (1.2675, -15.6822) ccw projected
  arc A28 (0.9858, -16.6417) -> (-0.9858, -16.6417) centre (0, -20) ccw projected
  arc A29 (-2.2662, -15.7322) -> (-0.9858, -16.6417) centre (-1.2675, -15.6822) ccw projected
  line L3 (-2.2662, -15.7322) -> (-2.4969, -11.125) projected
  arc A30 (2.4969, -11.125) -> (-2.4969, -11.125) centre (0, -11) ccw projected
  arc A31 (-6.5, 0) -> (-11.5307, 4.4686) centre (-11, 0) ccw
  arc A32 (-6.5, 0) -> (6.5, 0) centre (0, 0) ccw
  arc A33 (11.5307, 4.4686) -> (6.5, 0) centre (11, 0) ccw
  arc A34 (12.832, 3.234) -> (11.5307, 4.4686) centre (11.3538, 2.9791) ccw
  arc A35 (11.2015, 1.9898) -> (12.832, 3.234) centre (11.3527, 3.4822) ccw
  arc A36 (11.2015, 1.9898) -> (11.1178, -1.9965) centre (11, 0) ccw
  arc A37 (12.6381, -3.9404) -> (11.1178, -1.9965) centre (11.2061, -3.4939) ccw
  arc A38 (11.7228, -6.1502) -> (12.6381, -3.9404) centre (0, 0) ccw
  arc A39 (9.2732, -6.4497) -> (11.7228, -6.1502) centre (10.3945, -5.4533) ccw
  arc A40 (9.2732, -6.4497) -> (7.2312, -9.7019) centre (7.7782, -7.7782) ccw
  arc A41 (8.0864, -11.9501) -> (7.2312, -9.7019) centre (6.821, -11.1447) ccw
  line L4 (8.0864, -11.9501) -> (5.1463, -16.5699)
  arc A42 (5.1463, -16.5699) -> (4.4713, -19.493) centre (8.9427, -18.986) ccw
  arc A43 (-4.4713, -19.493) -> (4.4713, -19.493) centre (0, -20) ccw
  arc A44 (-4.4713, -19.493) -> (-5.1463, -16.5699) centre (-8.9427, -18.986) ccw
  line L5 (-5.1463, -16.5699) -> (-8.0864, -11.9501)
  arc A45 (-7.2312, -9.7019) -> (-8.0864, -11.9501) centre (-6.821, -11.1447) ccw
  arc A46 (-7.2312, -9.7019) -> (-9.2732, -6.4497) centre (-7.7782, -7.7782) ccw
  arc A47 (-11.7228, -6.1502) -> (-9.2732, -6.4497) centre (-10.3945, -5.4533) ccw
  arc A48 (-12.6381, -3.9404) -> (-11.7228, -6.1502) centre (0, 0) ccw
  arc A49 (-11.1178, -1.9965) -> (-12.6381, -3.9404) centre (-11.2061, -3.4939) ccw
  arc A50 (-11.1178, -1.9965) -> (-11.2015, 1.9898) centre (-11, 0) ccw
  arc A51 (-12.832, 3.234) -> (-11.2015, 1.9898) centre (-11.3527, 3.4822) ccw
  arc A52 (-11.5307, 4.4686) -> (-12.832, 3.234) centre (-11.3538, 2.9791) ccw
  point P0 (-12.3211, 3.2329)
  point P1 (12.3211, 3.2329)
  point P2 (11.4534, 4.4771)
  point P3 (-11.4534, 4.4771)
  dimension "d77" = 0.5
  constraints: 44 point on circle, 23 centre point, 4 end point, 2 coincident, 26 other
  measures "d77" radial gap between concentric circles of A24 A31
extrude "돌출21" add sketch "스케치22" against normal up to surface (5 mm away) contours A1 A24 A25 | A31 A32 A33 A3 A22 A23 A24 A1 | A3 A21 A22
sketch "스케치23" plane through (0, 0, 5) normal (0, 0, 1) x (1, 0, 0)
  arc A0 (-11.4534, 4.4771) -> (-11.2519, 2.4873) centre (-11.3527, 3.4822) ccw projected
  arc A1 (-11.1472, -2.4957) -> (-11.2519, 2.4873) centre (-11, 0) ccw projected
  arc A2 (-11.1472, -2.4957) -> (-12.1608, -3.7916) centre (-11.2061, -3.4939) ccw projected
  arc A3 (-12.1608, -3.7916) -> (-11.28, -5.9179) centre (0, 0) ccw projected
  arc A4 (-11.28, -5.9179) -> (-9.647, -6.1176) centre (-10.3945, -5.4533) ccw projected
  arc A5 (-7.0945, -10.1829) -> (-9.647, -6.1176) centre (-7.7782, -7.7782) ccw projected
  arc A6 (-7.0945, -10.1829) -> (-7.6646, -11.6816) centre (-6.821, -11.1447) ccw projected
  line L0 (-7.6646, -11.6816) -> (-4.7245, -16.3015) projected
  arc A7 (-3.9745, -19.5493) -> (-4.7245, -16.3015) centre (-8.9427, -18.986) ccw projected
  arc A8 (-3.9745, -19.5493) -> (3.9745, -19.5493) centre (0, -20) ccw projected
  arc A9 (4.7245, -16.3015) -> (3.9745, -19.5493) centre (8.9427, -18.986) ccw projected
  line L1 (4.7245, -16.3015) -> (7.6646, -11.6816) projected
  arc A10 (7.6646, -11.6816) -> (7.0945, -10.1829) centre (6.821, -11.1447) ccw projected
  arc A11 (9.647, -6.1176) -> (7.0945, -10.1829) centre (7.7782, -7.7782) ccw projected
  arc A12 (9.647, -6.1176) -> (11.28, -5.9179) centre (10.3945, -5.4533) ccw projected
  arc A13 (11.28, -5.9179) -> (12.1608, -3.7916) centre (0, 0) ccw projected
  arc A14 (12.1608, -3.7916) -> (11.1472, -2.4957) centre (11.2061, -3.4939) ccw projected
  arc A15 (11.2519, 2.4873) -> (11.1472, -2.4957) centre (11, 0) ccw projected
  arc A16 (11.2519, 2.4873) -> (11.4534, 4.4771) centre (11.3527, 3.4822) ccw projected
  arc A17 (11.4534, 4.4771) -> (6.5, 0) centre (11, 0) ccw projected
  arc A18 (-6.5, 0) -> (6.5, 0) centre (0, 0) ccw projected
  arc A19 (-6.5, 0) -> (-11.4534, 4.4771) centre (-11, 0) ccw projected
  circle A20 centre (0, -20) radius 2.05 projected
  line L2 (2.4969, -11.125) -> (2.2662, -15.7322) projected
  arc A21 (0.9858, -16.6417) -> (2.2662, -15.7322) centre (1.2675, -15.6822) ccw projected
  arc A22 (0.9858, -16.6417) -> (-0.9858, -16.6417) centre (0, -20) ccw projected
  arc A23 (-2.2662, -15.7322) -> (-0.9858, -16.6417) centre (-1.2675, -15.6822) ccw projected
  line L3 (-2.2662, -15.7322) -> (-2.4969, -11.125) projected
  arc A24 (2.4969, -11.125) -> (-2.4969, -11.125) centre (0, -11) ccw projected
  circle A25 centre (0, 0) radius 12.7381
  point P0 (12.0147, 4.2316)
  point P1 (12.3211, 3.2329)
  point P2 (-12.3211, 3.2329)
  point P3 (-12.0147, 4.2316)
  constraints: 1 centre point, 1 coincident, 1 concentric
extrude "돌출22" cut sketch "스케치23" against normal through all contours A25 A0 | A16 A25
fillet "모깎기5" radius 1 4 edges at (12.3211, 3.2329, 3.5) (12.0147, 4.2316, 2.5) (-12.3211, 3.2329, 3.5) (-12.0147, 4.2316, 2.5)
sketch "스케치24" plane through (0, 0, 5) normal (0, 0, 1) x (1, 0, 0)
  arc A0 (-11.265, 4.4922) -> (-11.1472, 2.4957) centre (-11.2061, 3.4939) ccw projected
  arc A1 (-11.1472, -2.4957) -> (-11.1472, 2.4957) centre (-11, 0) ccw projected
  arc A2 (-11.1472, -2.4957) -> (-12.1608, -3.7916) centre (-11.2061, -3.4939) ccw projected
  arc A3 (-12.1608, -3.7916) -> (-11.28, -5.9179) centre (0, 0) ccw projected
  arc A4 (-11.28, -5.9179) -> (-9.647, -6.1176) centre (-10.3945, -5.4533) ccw projected
  arc A5 (-7.0945, -10.1829) -> (-9.647, -6.1176) centre (-7.7782, -7.7782) ccw projected
  arc A6 (-7.0945, -10.1829) -> (-7.6646, -11.6816) centre (-6.821, -11.1447) ccw projected
  line L0 (-7.6646, -11.6816) -> (-4.7245, -16.3015) projected
  arc A7 (-3.9745, -19.5493) -> (-4.7245, -16.3015) centre (-8.9427, -18.986) ccw projected
  arc A8 (-3.9745, -19.5493) -> (3.9745, -19.5493) centre (0, -20) ccw projected
  arc A9 (4.7245, -16.3015) -> (3.9745, -19.5493) centre (8.9427, -18.986) ccw projected
  line L1 (4.7245, -16.3015) -> (7.6646, -11.6816) projected
  arc A10 (7.6646, -11.6816) -> (7.0945, -10.1829) centre (6.821, -11.1447) ccw projected
  arc A11 (9.647, -6.1176) -> (7.0945, -10.1829) centre (7.7782, -7.7782) ccw projected
  arc A12 (9.647, -6.1176) -> (11.28, -5.9179) centre (10.3945, -5.4533) ccw projected
  arc A13 (11.28, -5.9179) -> (12.1608, -3.7916) centre (0, 0) ccw projected
  arc A14 (12.1608, -3.7916) -> (11.1472, -2.4957) centre (11.2061, -3.4939) ccw projected
  arc A15 (11.1472, 2.4957) -> (11.1472, -2.4957) centre (11, 0) ccw projected
  arc A16 (11.1472, 2.4957) -> (11.265, 4.4922) centre (11.2061, 3.4939) ccw projected
  arc A17 (11.265, 4.4922) -> (6.5, 0) centre (11, 0) ccw projected
  arc A18 (-6.5, 0) -> (6.5, 0) centre (0, 0) ccw projected
  arc A19 (-6.5, 0) -> (-11.265, 4.4922) centre (-11, 0) ccw projected
  circle A20 centre (0, -20) radius 2.05 projected
  line L2 (2.4969, -11.125) -> (2.2662, -15.7322) projected
  arc A21 (0.9858, -16.6417) -> (2.2662, -15.7322) centre (1.2675, -15.6822) ccw projected
  arc A22 (0.9858, -16.6417) -> (-0.9858, -16.6417) centre (0, -20) ccw projected
  arc A23 (-2.2662, -15.7322) -> (-0.9858, -16.6417) centre (-1.2675, -15.6822) ccw projected
  line L3 (-2.2662, -15.7322) -> (-2.4969, -11.125) projected
  arc A24 (2.4969, -11.125) -> (-2.4969, -11.125) centre (0, -11) ccw projected
extrude "돌출23" cut sketch "스케치24" against normal blind 2